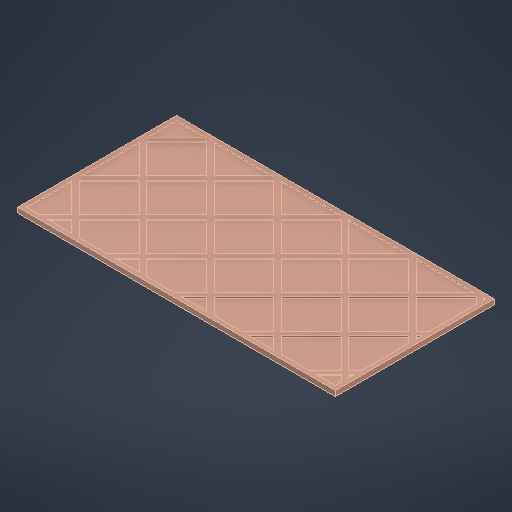
# Autodesk Inventor part: TILE 30X60
Saved by Autodesk Inventor 2025 (Build 290162000, 162)
## iProperties
Created: 2024-05-06
Part Number: TILE 30X60
Material: Generic
Document SubType Name: Modeling
Designer: zulet
Density: 1 g/cm^3
Appearance: Smooth - Dark Brown
Author: zulet
Autodesk Inventor part; units mm, degrees
ref_plane "YZ Plane" through (0, 0, 0) normal (1, 0, 0) x (0, 1, 0)
ref_plane "XZ Plane" through (0, 0, 0) normal (0, 1, 0) x (-1, 0, 0)
ref_plane "XY Plane" through (0, 0, 0) normal (0, 0, 1) x (1, 0, 0)
sketch "Sketch1" plane through (0, 0, 0) normal (0, 1, 0) x (-1, 0, 0)
  line L0 (0, 0) -> (600, 0)
  line L1 (600, 0) -> (600, -300)
  line L2 (600, -300) -> (0, -300)
  line L3 (0, -300) -> (0, 0)
  dimension "d0" = 600
  dimension "d1" = 300
  constraints: 8 end point, 2 parallel, 1 horizontal, 1 perpendicular
  measures "d0" distance of L1.end L2.end
  measures "d1" distance of L0.end L1.end
extrude "Extrusion1" add sketch "Sketch1" along normal blind 8
sketch "Sketch2" plane through (0, 8, 0) normal (0, 1, 0) x (1, 0, 0)
  line L0 (-656.5685, 300) -> (-600, 356.5685)
  line L1 (-600, 356.5685) -> (-656.5685, 413.1371)
  line L2 (-656.5685, 413.1371) -> (-713.1371, 356.5685)
  line L3 (-713.1371, 356.5685) -> (-656.5685, 300)
  line L4 (-656.5685, 300) -> (-656.5685, 413.1371) construction
  line L5 (-600, 356.5685) -> (-713.1371, 356.5685) construction
  line L6 (-656.5685, 300) -> (-576.5685, 300) construction
  line L7 (0, 300) -> (-600, 300) projected
  line L8 (-600, 300) -> (-600, 0) projected
  line L9 (-592.9289, 236.3604) -> (-536.3604, 292.9289)
  line L10 (-536.3604, 292.9289) -> (-592.9289, 349.4975)
  line L11 (-592.9289, 349.4975) -> (-649.4975, 292.9289)
  line L12 (-649.4975, 292.9289) -> (-592.9289, 236.3604)
  line L13 (-592.9289, 236.3604) -> (-592.9289, 349.4975) construction
  line L14 (-536.3604, 292.9289) -> (-649.4975, 292.9289) construction
  line L15 (-529.2893, 172.7208) -> (-472.7208, 229.2893)
  line L16 (-472.7208, 229.2893) -> (-529.2893, 285.8579)
  line L17 (-529.2893, 285.8579) -> (-585.8579, 229.2893)
  line L18 (-585.8579, 229.2893) -> (-529.2893, 172.7208)
  line L19 (-529.2893, 172.7208) -> (-529.2893, 285.8579) construction
  line L20 (-472.7208, 229.2893) -> (-585.8579, 229.2893) construction
  line L21 (-465.6497, 109.0812) -> (-409.0812, 165.6497)
  line L22 (-409.0812, 165.6497) -> (-465.6497, 222.2183)
  line L23 (-465.6497, 222.2183) -> (-522.2183, 165.6497)
  line L24 (-522.2183, 165.6497) -> (-465.6497, 109.0812)
  line L25 (-465.6497, 109.0812) -> (-465.6497, 222.2183) construction
  line L26 (-409.0812, 165.6497) -> (-522.2183, 165.6497) construction
  line L27 (-402.0101, 45.4416) -> (-345.4416, 102.0101)
  line L28 (-345.4416, 102.0101) -> (-402.0101, 158.5786)
  line L29 (-402.0101, 158.5786) -> (-458.5786, 102.0101)
  line L30 (-458.5786, 102.0101) -> (-402.0101, 45.4416)
  line L31 (-402.0101, 45.4416) -> (-402.0101, 158.5786) construction
  line L32 (-345.4416, 102.0101) -> (-458.5786, 102.0101) construction
  line L33 (-338.3705, -18.1981) -> (-281.8019, 38.3705)
  line L34 (-281.8019, 38.3705) -> (-338.3705, 94.939)
  line L35 (-338.3705, 94.939) -> (-394.939, 38.3705)
  line L36 (-394.939, 38.3705) -> (-338.3705, -18.1981)
  line L37 (-338.3705, -18.1981) -> (-338.3705, 94.939) construction
  line L38 (-281.8019, 38.3705) -> (-394.939, 38.3705) construction
  line L39 (-274.7309, -81.8377) -> (-218.1623, -25.2691)
  line L40 (-218.1623, -25.2691) -> (-274.7309, 31.2994)
  line L41 (-274.7309, 31.2994) -> (-331.2994, -25.2691)
  line L42 (-331.2994, -25.2691) -> (-274.7309, -81.8377)
  line L43 (-274.7309, -81.8377) -> (-274.7309, 31.2994) construction
  line L44 (-218.1623, -25.2691) -> (-331.2994, -25.2691) construction
  line L45 (-211.0913, -145.4773) -> (-154.5227, -88.9087)
  line L46 (-154.5227, -88.9087) -> (-211.0913, -32.3402)
  line L47 (-211.0913, -32.3402) -> (-267.6598, -88.9087)
  line L48 (-267.6598, -88.9087) -> (-211.0913, -145.4773)
  line L49 (-211.0913, -145.4773) -> (-211.0913, -32.3402) construction
  line L50 (-154.5227, -88.9087) -> (-267.6598, -88.9087) construction
  line L51 (-147.4517, -209.1169) -> (-90.8831, -152.5483)
  line L52 (-90.8831, -152.5483) -> (-147.4517, -95.9798)
  line L53 (-147.4517, -95.9798) -> (-204.0202, -152.5483)
  line L54 (-204.0202, -152.5483) -> (-147.4517, -209.1169)
  line L55 (-147.4517, -209.1169) -> (-147.4517, -95.9798) construction
  line L56 (-90.8831, -152.5483) -> (-204.0202, -152.5483) construction
  line L57 (-83.812, -272.7565) -> (-27.2435, -216.188)
  line L58 (-27.2435, -216.188) -> (-83.812, -159.6194)
  line L59 (-83.812, -159.6194) -> (-140.3806, -216.188)
  line L60 (-140.3806, -216.188) -> (-83.812, -272.7565)
  line L61 (-83.812, -272.7565) -> (-83.812, -159.6194) construction
  line L62 (-27.2435, -216.188) -> (-140.3806, -216.188) construction
  line L63 (-592.9289, 363.6396) -> (-536.3604, 420.2082)
  line L64 (-536.3604, 420.2082) -> (-592.9289, 476.7767)
  line L65 (-592.9289, 476.7767) -> (-649.4975, 420.2082)
  line L66 (-649.4975, 420.2082) -> (-592.9289, 363.6396)
  line L67 (-592.9289, 363.6396) -> (-592.9289, 476.7767) construction
  line L68 (-536.3604, 420.2082) -> (-649.4975, 420.2082) construction
  line L69 (-529.2893, 300) -> (-472.7208, 356.5685)
  line L70 (-472.7208, 356.5685) -> (-529.2893, 413.1371)
  line L71 (-529.2893, 413.1371) -> (-585.8579, 356.5685)
  line L72 (-585.8579, 356.5685) -> (-529.2893, 300)
  line L73 (-529.2893, 300) -> (-529.2893, 413.1371) construction
  line L74 (-472.7208, 356.5685) -> (-585.8579, 356.5685) construction
  line L75 (-465.6497, 236.3604) -> (-409.0812, 292.9289)
  line L76 (-409.0812, 292.9289) -> (-465.6497, 349.4975)
  line L77 (-465.6497, 349.4975) -> (-522.2183, 292.9289)
  line L78 (-522.2183, 292.9289) -> (-465.6497, 236.3604)
  line L79 (-465.6497, 236.3604) -> (-465.6497, 349.4975) construction
  line L80 (-409.0812, 292.9289) -> (-522.2183, 292.9289) construction
  line L81 (-402.0101, 172.7208) -> (-345.4416, 229.2893)
  line L82 (-345.4416, 229.2893) -> (-402.0101, 285.8579)
  line L83 (-402.0101, 285.8579) -> (-458.5786, 229.2893)
  line L84 (-458.5786, 229.2893) -> (-402.0101, 172.7208)
  line L85 (-402.0101, 172.7208) -> (-402.0101, 285.8579) construction
  line L86 (-345.4416, 229.2893) -> (-458.5786, 229.2893) construction
  line L87 (-338.3705, 109.0812) -> (-281.8019, 165.6497)
  line L88 (-281.8019, 165.6497) -> (-338.3705, 222.2183)
  line L89 (-338.3705, 222.2183) -> (-394.939, 165.6497)
  line L90 (-394.939, 165.6497) -> (-338.3705, 109.0812)
  line L91 (-338.3705, 109.0812) -> (-338.3705, 222.2183) construction
  line L92 (-281.8019, 165.6497) -> (-394.939, 165.6497) construction
  line L93 (-274.7309, 45.4416) -> (-218.1623, 102.0101)
  line L94 (-218.1623, 102.0101) -> (-274.7309, 158.5786)
  line L95 (-274.7309, 158.5786) -> (-331.2994, 102.0101)
  line L96 (-331.2994, 102.0101) -> (-274.7309, 45.4416)
  line L97 (-274.7309, 45.4416) -> (-274.7309, 158.5786) construction
  line L98 (-218.1623, 102.0101) -> (-331.2994, 102.0101) construction
  line L99 (-211.0913, -18.1981) -> (-154.5227, 38.3705)
  line L100 (-154.5227, 38.3705) -> (-211.0913, 94.939)
  line L101 (-211.0913, 94.939) -> (-267.6598, 38.3705)
  line L102 (-267.6598, 38.3705) -> (-211.0913, -18.1981)
  line L103 (-211.0913, -18.1981) -> (-211.0913, 94.939) construction
  line L104 (-154.5227, 38.3705) -> (-267.6598, 38.3705) construction
  line L105 (-147.4517, -81.8377) -> (-90.8831, -25.2691)
  line L106 (-90.8831, -25.2691) -> (-147.4517, 31.2994)
  line L107 (-147.4517, 31.2994) -> (-204.0202, -25.2691)
  line L108 (-204.0202, -25.2691) -> (-147.4517, -81.8377)
  line L109 (-147.4517, -81.8377) -> (-147.4517, 31.2994) construction
  line L110 (-90.8831, -25.2691) -> (-204.0202, -25.2691) construction
  line L111 (-83.812, -145.4773) -> (-27.2435, -88.9087)
  line L112 (-27.2435, -88.9087) -> (-83.812, -32.3402)
  line L113 (-83.812, -32.3402) -> (-140.3806, -88.9087)
  line L114 (-140.3806, -88.9087) -> (-83.812, -145.4773)
  line L115 (-83.812, -145.4773) -> (-83.812, -32.3402) construction
  line L116 (-27.2435, -88.9087) -> (-140.3806, -88.9087) construction
  line L117 (-20.1724, -209.1169) -> (36.3961, -152.5483)
  line L118 (36.3961, -152.5483) -> (-20.1724, -95.9798)
  line L119 (-20.1724, -95.9798) -> (-76.741, -152.5483)
  line L120 (-76.741, -152.5483) -> (-20.1724, -209.1169)
  line L121 (-20.1724, -209.1169) -> (-20.1724, -95.9798) construction
  line L122 (36.3961, -152.5483) -> (-76.741, -152.5483) construction
  line L123 (-720.2082, 236.3604) -> (-663.6396, 292.9289)
  line L124 (-663.6396, 292.9289) -> (-720.2082, 349.4975)
  line L125 (-720.2082, 349.4975) -> (-776.7767, 292.9289)
  line L126 (-776.7767, 292.9289) -> (-720.2082, 236.3604)
  line L127 (-720.2082, 236.3604) -> (-720.2082, 349.4975) construction
  line L128 (-663.6396, 292.9289) -> (-776.7767, 292.9289) construction
  line L129 (-656.5685, 172.7208) -> (-600, 229.2893)
  line L130 (-600, 229.2893) -> (-656.5685, 285.8579)
  line L131 (-656.5685, 285.8579) -> (-713.1371, 229.2893)
  line L132 (-713.1371, 229.2893) -> (-656.5685, 172.7208)
  line L133 (-656.5685, 172.7208) -> (-656.5685, 285.8579) construction
  line L134 (-600, 229.2893) -> (-713.1371, 229.2893) construction
  line L135 (-592.9289, 109.0812) -> (-536.3604, 165.6497)
  line L136 (-536.3604, 165.6497) -> (-592.9289, 222.2183)
  line L137 (-592.9289, 222.2183) -> (-649.4975, 165.6497)
  line L138 (-649.4975, 165.6497) -> (-592.9289, 109.0812)
  line L139 (-592.9289, 109.0812) -> (-592.9289, 222.2183) construction
  line L140 (-536.3604, 165.6497) -> (-649.4975, 165.6497) construction
  line L141 (-529.2893, 45.4416) -> (-472.7208, 102.0101)
  line L142 (-472.7208, 102.0101) -> (-529.2893, 158.5786)
  line L143 (-529.2893, 158.5786) -> (-585.8579, 102.0101)
  line L144 (-585.8579, 102.0101) -> (-529.2893, 45.4416)
  line L145 (-529.2893, 45.4416) -> (-529.2893, 158.5786) construction
  line L146 (-472.7208, 102.0101) -> (-585.8579, 102.0101) construction
  line L147 (-465.6497, -18.1981) -> (-409.0812, 38.3705)
  line L148 (-409.0812, 38.3705) -> (-465.6497, 94.939)
  line L149 (-465.6497, 94.939) -> (-522.2183, 38.3705)
  line L150 (-522.2183, 38.3705) -> (-465.6497, -18.1981)
  line L151 (-465.6497, -18.1981) -> (-465.6497, 94.939) construction
  line L152 (-409.0812, 38.3705) -> (-522.2183, 38.3705) construction
  line L153 (-402.0101, -81.8377) -> (-345.4416, -25.2691)
  line L154 (-345.4416, -25.2691) -> (-402.0101, 31.2994)
  line L155 (-402.0101, 31.2994) -> (-458.5786, -25.2691)
  line L156 (-458.5786, -25.2691) -> (-402.0101, -81.8377)
  line L157 (-402.0101, -81.8377) -> (-402.0101, 31.2994) construction
  line L158 (-345.4416, -25.2691) -> (-458.5786, -25.2691) construction
  line L159 (-338.3705, -145.4773) -> (-281.8019, -88.9087)
  line L160 (-281.8019, -88.9087) -> (-338.3705, -32.3402)
  line L161 (-338.3705, -32.3402) -> (-394.939, -88.9087)
  line L162 (-394.939, -88.9087) -> (-338.3705, -145.4773)
  line L163 (-338.3705, -145.4773) -> (-338.3705, -32.3402) construction
  line L164 (-281.8019, -88.9087) -> (-394.939, -88.9087) construction
  line L165 (-274.7309, -209.1169) -> (-218.1623, -152.5483)
  line L166 (-218.1623, -152.5483) -> (-274.7309, -95.9798)
  line L167 (-274.7309, -95.9798) -> (-331.2994, -152.5483)
  line L168 (-331.2994, -152.5483) -> (-274.7309, -209.1169)
  line L169 (-274.7309, -209.1169) -> (-274.7309, -95.9798) construction
  line L170 (-218.1623, -152.5483) -> (-331.2994, -152.5483) construction
  line L171 (-211.0913, -272.7565) -> (-154.5227, -216.188)
  line L172 (-154.5227, -216.188) -> (-211.0913, -159.6194)
  line L173 (-211.0913, -159.6194) -> (-267.6598, -216.188)
  line L174 (-267.6598, -216.188) -> (-211.0913, -272.7565)
  line L175 (-211.0913, -272.7565) -> (-211.0913, -159.6194) construction
  line L176 (-154.5227, -216.188) -> (-267.6598, -216.188) construction
  line L177 (-147.4517, -336.3961) -> (-90.8831, -279.8276)
  line L178 (-90.8831, -279.8276) -> (-147.4517, -223.259)
  line L179 (-147.4517, -223.259) -> (-204.0202, -279.8276)
  line L180 (-204.0202, -279.8276) -> (-147.4517, -336.3961)
  line L181 (-147.4517, -336.3961) -> (-147.4517, -223.259) construction
  line L182 (-90.8831, -279.8276) -> (-204.0202, -279.8276) construction
  line L183 (-529.2893, 427.2792) -> (-472.7208, 483.8478)
  line L184 (-472.7208, 483.8478) -> (-529.2893, 540.4163)
  line L185 (-529.2893, 540.4163) -> (-585.8579, 483.8478)
  line L186 (-585.8579, 483.8478) -> (-529.2893, 427.2792)
  line L187 (-529.2893, 427.2792) -> (-529.2893, 540.4163) construction
  line L188 (-472.7208, 483.8478) -> (-585.8579, 483.8478) construction
  line L189 (-465.6497, 363.6396) -> (-409.0812, 420.2082)
  line L190 (-409.0812, 420.2082) -> (-465.6497, 476.7767)
  line L191 (-465.6497, 476.7767) -> (-522.2183, 420.2082)
  line L192 (-522.2183, 420.2082) -> (-465.6497, 363.6396)
  line L193 (-465.6497, 363.6396) -> (-465.6497, 476.7767) construction
  line L194 (-409.0812, 420.2082) -> (-522.2183, 420.2082) construction
  line L195 (-402.0101, 300) -> (-345.4416, 356.5685)
  line L196 (-345.4416, 356.5685) -> (-402.0101, 413.1371)
  line L197 (-402.0101, 413.1371) -> (-458.5786, 356.5685)
  line L198 (-458.5786, 356.5685) -> (-402.0101, 300)
  line L199 (-402.0101, 300) -> (-402.0101, 413.1371) construction
  line L200 (-345.4416, 356.5685) -> (-458.5786, 356.5685) construction
  line L201 (-338.3705, 236.3604) -> (-281.8019, 292.9289)
  line L202 (-281.8019, 292.9289) -> (-338.3705, 349.4975)
  line L203 (-338.3705, 349.4975) -> (-394.939, 292.9289)
  line L204 (-394.939, 292.9289) -> (-338.3705, 236.3604)
  line L205 (-338.3705, 236.3604) -> (-338.3705, 349.4975) construction
  line L206 (-281.8019, 292.9289) -> (-394.939, 292.9289) construction
  line L207 (-274.7309, 172.7208) -> (-218.1623, 229.2893)
  line L208 (-218.1623, 229.2893) -> (-274.7309, 285.8579)
  line L209 (-274.7309, 285.8579) -> (-331.2994, 229.2893)
  line L210 (-331.2994, 229.2893) -> (-274.7309, 172.7208)
  line L211 (-274.7309, 172.7208) -> (-274.7309, 285.8579) construction
  line L212 (-218.1623, 229.2893) -> (-331.2994, 229.2893) construction
  line L213 (-211.0913, 109.0812) -> (-154.5227, 165.6497)
  line L214 (-154.5227, 165.6497) -> (-211.0913, 222.2183)
  line L215 (-211.0913, 222.2183) -> (-267.6598, 165.6497)
  line L216 (-267.6598, 165.6497) -> (-211.0913, 109.0812)
  line L217 (-211.0913, 109.0812) -> (-211.0913, 222.2183) construction
  line L218 (-154.5227, 165.6497) -> (-267.6598, 165.6497) construction
  line L219 (-147.4517, 45.4416) -> (-90.8831, 102.0101)
  line L220 (-90.8831, 102.0101) -> (-147.4517, 158.5786)
  line L221 (-147.4517, 158.5786) -> (-204.0202, 102.0101)
  line L222 (-204.0202, 102.0101) -> (-147.4517, 45.4416)
  line L223 (-147.4517, 45.4416) -> (-147.4517, 158.5786) construction
  line L224 (-90.8831, 102.0101) -> (-204.0202, 102.0101) construction
  line L225 (-83.812, -18.1981) -> (-27.2435, 38.3705)
  line L226 (-27.2435, 38.3705) -> (-83.812, 94.939)
  line L227 (-83.812, 94.939) -> (-140.3806, 38.3705)
  line L228 (-140.3806, 38.3705) -> (-83.812, -18.1981)
  line L229 (-83.812, -18.1981) -> (-83.812, 94.939) construction
  line L230 (-27.2435, 38.3705) -> (-140.3806, 38.3705) construction
  line L231 (-20.1724, -81.8377) -> (36.3961, -25.2691)
  line L232 (36.3961, -25.2691) -> (-20.1724, 31.2994)
  line L233 (-20.1724, 31.2994) -> (-76.741, -25.2691)
  line L234 (-76.741, -25.2691) -> (-20.1724, -81.8377)
  line L235 (-20.1724, -81.8377) -> (-20.1724, 31.2994) construction
  line L236 (36.3961, -25.2691) -> (-76.741, -25.2691) construction
  line L237 (43.4672, -145.4773) -> (100.0357, -88.9087)
  line L238 (100.0357, -88.9087) -> (43.4672, -32.3402)
  line L239 (43.4672, -32.3402) -> (-13.1014, -88.9087)
  line L240 (-13.1014, -88.9087) -> (43.4672, -145.4773)
  line L241 (43.4672, -145.4773) -> (43.4672, -32.3402) construction
  line L242 (100.0357, -88.9087) -> (-13.1014, -88.9087) construction
  line L243 (-783.8478, 172.7208) -> (-727.2792, 229.2893)
  line L244 (-727.2792, 229.2893) -> (-783.8478, 285.8579)
  line L245 (-783.8478, 285.8579) -> (-840.4163, 229.2893)
  line L246 (-840.4163, 229.2893) -> (-783.8478, 172.7208)
  line L247 (-783.8478, 172.7208) -> (-783.8478, 285.8579) construction
  line L248 (-727.2792, 229.2893) -> (-840.4163, 229.2893) construction
  line L249 (-720.2082, 109.0812) -> (-663.6396, 165.6497)
  line L250 (-663.6396, 165.6497) -> (-720.2082, 222.2183)
  line L251 (-720.2082, 222.2183) -> (-776.7767, 165.6497)
  line L252 (-776.7767, 165.6497) -> (-720.2082, 109.0812)
  line L253 (-720.2082, 109.0812) -> (-720.2082, 222.2183) construction
  line L254 (-663.6396, 165.6497) -> (-776.7767, 165.6497) construction
  line L255 (-656.5685, 45.4416) -> (-600, 102.0101)
  line L256 (-600, 102.0101) -> (-656.5685, 158.5786)
  line L257 (-656.5685, 158.5786) -> (-713.1371, 102.0101)
  line L258 (-713.1371, 102.0101) -> (-656.5685, 45.4416)
  line L259 (-656.5685, 45.4416) -> (-656.5685, 158.5786) construction
  line L260 (-600, 102.0101) -> (-713.1371, 102.0101) construction
  line L261 (-592.9289, -18.1981) -> (-536.3604, 38.3705)
  line L262 (-536.3604, 38.3705) -> (-592.9289, 94.939)
  line L263 (-592.9289, 94.939) -> (-649.4975, 38.3705)
  line L264 (-649.4975, 38.3705) -> (-592.9289, -18.1981)
  line L265 (-592.9289, -18.1981) -> (-592.9289, 94.939) construction
  line L266 (-536.3604, 38.3705) -> (-649.4975, 38.3705) construction
  line L267 (-529.2893, -81.8377) -> (-472.7208, -25.2691)
  line L268 (-472.7208, -25.2691) -> (-529.2893, 31.2994)
  line L269 (-529.2893, 31.2994) -> (-585.8579, -25.2691)
  line L270 (-585.8579, -25.2691) -> (-529.2893, -81.8377)
  line L271 (-529.2893, -81.8377) -> (-529.2893, 31.2994) construction
  line L272 (-472.7208, -25.2691) -> (-585.8579, -25.2691) construction
  line L273 (-465.6497, -145.4773) -> (-409.0812, -88.9087)
  line L274 (-409.0812, -88.9087) -> (-465.6497, -32.3402)
  line L275 (-465.6497, -32.3402) -> (-522.2183, -88.9087)
  line L276 (-522.2183, -88.9087) -> (-465.6497, -145.4773)
  line L277 (-465.6497, -145.4773) -> (-465.6497, -32.3402) construction
  line L278 (-409.0812, -88.9087) -> (-522.2183, -88.9087) construction
  line L279 (-402.0101, -209.1169) -> (-345.4416, -152.5483)
  line L280 (-345.4416, -152.5483) -> (-402.0101, -95.9798)
  line L281 (-402.0101, -95.9798) -> (-458.5786, -152.5483)
  line L282 (-458.5786, -152.5483) -> (-402.0101, -209.1169)
  line L283 (-402.0101, -209.1169) -> (-402.0101, -95.9798) construction
  line L284 (-345.4416, -152.5483) -> (-458.5786, -152.5483) construction
  line L285 (-338.3705, -272.7565) -> (-281.8019, -216.188)
  line L286 (-281.8019, -216.188) -> (-338.3705, -159.6194)
  line L287 (-338.3705, -159.6194) -> (-394.939, -216.188)
  line L288 (-394.939, -216.188) -> (-338.3705, -272.7565)
  line L289 (-338.3705, -272.7565) -> (-338.3705, -159.6194) construction
  line L290 (-281.8019, -216.188) -> (-394.939, -216.188) construction
  line L291 (-274.7309, -336.3961) -> (-218.1623, -279.8276)
  line L292 (-218.1623, -279.8276) -> (-274.7309, -223.259)
  line L293 (-274.7309, -223.259) -> (-331.2994, -279.8276)
  line L294 (-331.2994, -279.8276) -> (-274.7309, -336.3961)
  line L295 (-274.7309, -336.3961) -> (-274.7309, -223.259) construction
  line L296 (-218.1623, -279.8276) -> (-331.2994, -279.8276) construction
  line L297 (-211.0913, -400.0357) -> (-154.5227, -343.4672)
  line L298 (-154.5227, -343.4672) -> (-211.0913, -286.8986)
  line L299 (-211.0913, -286.8986) -> (-267.6598, -343.4672)
  line L300 (-267.6598, -343.4672) -> (-211.0913, -400.0357)
  line L301 (-211.0913, -400.0357) -> (-211.0913, -286.8986) construction
  line L302 (-154.5227, -343.4672) -> (-267.6598, -343.4672) construction
  line L303 (-465.6497, 490.9188) -> (-409.0812, 547.4874)
  line L304 (-409.0812, 547.4874) -> (-465.6497, 604.0559)
  line L305 (-465.6497, 604.0559) -> (-522.2183, 547.4874)
  line L306 (-522.2183, 547.4874) -> (-465.6497, 490.9188)
  line L307 (-465.6497, 490.9188) -> (-465.6497, 604.0559) construction
  line L308 (-409.0812, 547.4874) -> (-522.2183, 547.4874) construction
  line L309 (-402.0101, 427.2792) -> (-345.4416, 483.8478)
  line L310 (-345.4416, 483.8478) -> (-402.0101, 540.4163)
  line L311 (-402.0101, 540.4163) -> (-458.5786, 483.8478)
  line L312 (-458.5786, 483.8478) -> (-402.0101, 427.2792)
  line L313 (-402.0101, 427.2792) -> (-402.0101, 540.4163) construction
  line L314 (-345.4416, 483.8478) -> (-458.5786, 483.8478) construction
  line L315 (-338.3705, 363.6396) -> (-281.8019, 420.2082)
  line L316 (-281.8019, 420.2082) -> (-338.3705, 476.7767)
  line L317 (-338.3705, 476.7767) -> (-394.939, 420.2082)
  line L318 (-394.939, 420.2082) -> (-338.3705, 363.6396)
  line L319 (-338.3705, 363.6396) -> (-338.3705, 476.7767) construction
  line L320 (-281.8019, 420.2082) -> (-394.939, 420.2082) construction
  line L321 (-274.7309, 300) -> (-218.1623, 356.5685)
  line L322 (-218.1623, 356.5685) -> (-274.7309, 413.1371)
  line L323 (-274.7309, 413.1371) -> (-331.2994, 356.5685)
  line L324 (-331.2994, 356.5685) -> (-274.7309, 300)
  line L325 (-274.7309, 300) -> (-274.7309, 413.1371) construction
  line L326 (-218.1623, 356.5685) -> (-331.2994, 356.5685) construction
  line L327 (-211.0913, 236.3604) -> (-154.5227, 292.9289)
  line L328 (-154.5227, 292.9289) -> (-211.0913, 349.4975)
  line L329 (-211.0913, 349.4975) -> (-267.6598, 292.9289)
  line L330 (-267.6598, 292.9289) -> (-211.0913, 236.3604)
  line L331 (-211.0913, 236.3604) -> (-211.0913, 349.4975) construction
  line L332 (-154.5227, 292.9289) -> (-267.6598, 292.9289) construction
  line L333 (-147.4517, 172.7208) -> (-90.8831, 229.2893)
  line L334 (-90.8831, 229.2893) -> (-147.4517, 285.8579)
  line L335 (-147.4517, 285.8579) -> (-204.0202, 229.2893)
  line L336 (-204.0202, 229.2893) -> (-147.4517, 172.7208)
  line L337 (-147.4517, 172.7208) -> (-147.4517, 285.8579) construction
  line L338 (-90.8831, 229.2893) -> (-204.0202, 229.2893) construction
  line L339 (-83.812, 109.0812) -> (-27.2435, 165.6497)
  line L340 (-27.2435, 165.6497) -> (-83.812, 222.2183)
  line L341 (-83.812, 222.2183) -> (-140.3806, 165.6497)
  line L342 (-140.3806, 165.6497) -> (-83.812, 109.0812)
  line L343 (-83.812, 109.0812) -> (-83.812, 222.2183) construction
  line L344 (-27.2435, 165.6497) -> (-140.3806, 165.6497) construction
  line L345 (-20.1724, 45.4416) -> (36.3961, 102.0101)
  line L346 (36.3961, 102.0101) -> (-20.1724, 158.5786)
  line L347 (-20.1724, 158.5786) -> (-76.741, 102.0101)
  line L348 (-76.741, 102.0101) -> (-20.1724, 45.4416)
  line L349 (-20.1724, 45.4416) -> (-20.1724, 158.5786) construction
  line L350 (36.3961, 102.0101) -> (-76.741, 102.0101) construction
  line L351 (43.4672, -18.1981) -> (100.0357, 38.3705)
  line L352 (100.0357, 38.3705) -> (43.4672, 94.939)
  line L353 (43.4672, 94.939) -> (-13.1014, 38.3705)
  line L354 (-13.1014, 38.3705) -> (43.4672, -18.1981)
  line L355 (43.4672, -18.1981) -> (43.4672, 94.939) construction
  line L356 (100.0357, 38.3705) -> (-13.1014, 38.3705) construction
  line L357 (107.1068, -81.8377) -> (163.6753, -25.2691)
  line L358 (163.6753, -25.2691) -> (107.1068, 31.2994)
  line L359 (107.1068, 31.2994) -> (50.5382, -25.2691)
  line L360 (50.5382, -25.2691) -> (107.1068, -81.8377)
  line L361 (107.1068, -81.8377) -> (107.1068, 31.2994) construction
  line L362 (163.6753, -25.2691) -> (50.5382, -25.2691) construction
  line L363 (-847.4874, 109.0812) -> (-790.9188, 165.6497)
  line L364 (-790.9188, 165.6497) -> (-847.4874, 222.2183)
  line L365 (-847.4874, 222.2183) -> (-904.0559, 165.6497)
  line L366 (-904.0559, 165.6497) -> (-847.4874, 109.0812)
  line L367 (-847.4874, 109.0812) -> (-847.4874, 222.2183) construction
  line L368 (-790.9188, 165.6497) -> (-904.0559, 165.6497) construction
  line L369 (-783.8478, 45.4416) -> (-727.2792, 102.0101)
  line L370 (-727.2792, 102.0101) -> (-783.8478, 158.5786)
  line L371 (-783.8478, 158.5786) -> (-840.4163, 102.0101)
  line L372 (-840.4163, 102.0101) -> (-783.8478, 45.4416)
  line L373 (-783.8478, 45.4416) -> (-783.8478, 158.5786) construction
  line L374 (-727.2792, 102.0101) -> (-840.4163, 102.0101) construction
  line L375 (-720.2082, -18.1981) -> (-663.6396, 38.3705)
  line L376 (-663.6396, 38.3705) -> (-720.2082, 94.939)
  line L377 (-720.2082, 94.939) -> (-776.7767, 38.3705)
  line L378 (-776.7767, 38.3705) -> (-720.2082, -18.1981)
  line L379 (-720.2082, -18.1981) -> (-720.2082, 94.939) construction
  line L380 (-663.6396, 38.3705) -> (-776.7767, 38.3705) construction
  line L381 (-656.5685, -81.8377) -> (-600, -25.2691)
  line L382 (-600, -25.2691) -> (-656.5685, 31.2994)
  line L383 (-656.5685, 31.2994) -> (-713.1371, -25.2691)
  line L384 (-713.1371, -25.2691) -> (-656.5685, -81.8377)
  line L385 (-656.5685, -81.8377) -> (-656.5685, 31.2994) construction
  line L386 (-600, -25.2691) -> (-713.1371, -25.2691) construction
  line L387 (-592.9289, -145.4773) -> (-536.3604, -88.9087)
  line L388 (-536.3604, -88.9087) -> (-592.9289, -32.3402)
  line L389 (-592.9289, -32.3402) -> (-649.4975, -88.9087)
  line L390 (-649.4975, -88.9087) -> (-592.9289, -145.4773)
  line L391 (-592.9289, -145.4773) -> (-592.9289, -32.3402) construction
  line L392 (-536.3604, -88.9087) -> (-649.4975, -88.9087) construction
  line L393 (-529.2893, -209.1169) -> (-472.7208, -152.5483)
  line L394 (-472.7208, -152.5483) -> (-529.2893, -95.9798)
  line L395 (-529.2893, -95.9798) -> (-585.8579, -152.5483)
  line L396 (-585.8579, -152.5483) -> (-529.2893, -209.1169)
  line L397 (-529.2893, -209.1169) -> (-529.2893, -95.9798) construction
  line L398 (-472.7208, -152.5483) -> (-585.8579, -152.5483) construction
  line L399 (-465.6497, -272.7565) -> (-409.0812, -216.188)
  line L400 (-409.0812, -216.188) -> (-465.6497, -159.6194)
  line L401 (-465.6497, -159.6194) -> (-522.2183, -216.188)
  line L402 (-522.2183, -216.188) -> (-465.6497, -272.7565)
  line L403 (-465.6497, -272.7565) -> (-465.6497, -159.6194) construction
  line L404 (-409.0812, -216.188) -> (-522.2183, -216.188) construction
  line L405 (-402.0101, -336.3961) -> (-345.4416, -279.8276)
  line L406 (-345.4416, -279.8276) -> (-402.0101, -223.259)
  line L407 (-402.0101, -223.259) -> (-458.5786, -279.8276)
  line L408 (-458.5786, -279.8276) -> (-402.0101, -336.3961)
  line L409 (-402.0101, -336.3961) -> (-402.0101, -223.259) construction
  line L410 (-345.4416, -279.8276) -> (-458.5786, -279.8276) construction
  line L411 (-338.3705, -400.0357) -> (-281.8019, -343.4672)
  line L412 (-281.8019, -343.4672) -> (-338.3705, -286.8986)
  line L413 (-338.3705, -286.8986) -> (-394.939, -343.4672)
  line L414 (-394.939, -343.4672) -> (-338.3705, -400.0357)
  line L415 (-338.3705, -400.0357) -> (-338.3705, -286.8986) construction
  line L416 (-281.8019, -343.4672) -> (-394.939, -343.4672) construction
  line L417 (-274.7309, -463.6753) -> (-218.1623, -407.1068)
  line L418 (-218.1623, -407.1068) -> (-274.7309, -350.5382)
  line L419 (-274.7309, -350.5382) -> (-331.2994, -407.1068)
  line L420 (-331.2994, -407.1068) -> (-274.7309, -463.6753)
  line L421 (-274.7309, -463.6753) -> (-274.7309, -350.5382) construction
  line L422 (-218.1623, -407.1068) -> (-331.2994, -407.1068) construction
  line L423 (-402.0101, 554.5584) -> (-345.4416, 611.127)
  line L424 (-345.4416, 611.127) -> (-402.0101, 667.6955)
  line L425 (-402.0101, 667.6955) -> (-458.5786, 611.127)
  line L426 (-458.5786, 611.127) -> (-402.0101, 554.5584)
  line L427 (-402.0101, 554.5584) -> (-402.0101, 667.6955) construction
  line L428 (-345.4416, 611.127) -> (-458.5786, 611.127) construction
  line L429 (-338.3705, 490.9188) -> (-281.8019, 547.4874)
  line L430 (-281.8019, 547.4874) -> (-338.3705, 604.0559)
  line L431 (-338.3705, 604.0559) -> (-394.939, 547.4874)
  line L432 (-394.939, 547.4874) -> (-338.3705, 490.9188)
  line L433 (-338.3705, 490.9188) -> (-338.3705, 604.0559) construction
  line L434 (-281.8019, 547.4874) -> (-394.939, 547.4874) construction
  line L435 (-274.7309, 427.2792) -> (-218.1623, 483.8478)
  line L436 (-218.1623, 483.8478) -> (-274.7309, 540.4163)
  line L437 (-274.7309, 540.4163) -> (-331.2994, 483.8478)
  line L438 (-331.2994, 483.8478) -> (-274.7309, 427.2792)
  line L439 (-274.7309, 427.2792) -> (-274.7309, 540.4163) construction
  line L440 (-218.1623, 483.8478) -> (-331.2994, 483.8478) construction
  line L441 (-211.0913, 363.6396) -> (-154.5227, 420.2082)
  line L442 (-154.5227, 420.2082) -> (-211.0913, 476.7767)
  line L443 (-211.0913, 476.7767) -> (-267.6598, 420.2082)
  line L444 (-267.6598, 420.2082) -> (-211.0913, 363.6396)
  line L445 (-211.0913, 363.6396) -> (-211.0913, 476.7767) construction
  line L446 (-154.5227, 420.2082) -> (-267.6598, 420.2082) construction
  line L447 (-147.4517, 300) -> (-90.8831, 356.5685)
  line L448 (-90.8831, 356.5685) -> (-147.4517, 413.1371)
  line L449 (-147.4517, 413.1371) -> (-204.0202, 356.5685)
  line L450 (-204.0202, 356.5685) -> (-147.4517, 300)
  line L451 (-147.4517, 300) -> (-147.4517, 413.1371) construction
  line L452 (-90.8831, 356.5685) -> (-204.0202, 356.5685) construction
  line L453 (-83.812, 236.3604) -> (-27.2435, 292.9289)
  line L454 (-27.2435, 292.9289) -> (-83.812, 349.4975)
  line L455 (-83.812, 349.4975) -> (-140.3806, 292.9289)
  line L456 (-140.3806, 292.9289) -> (-83.812, 236.3604)
  line L457 (-83.812, 236.3604) -> (-83.812, 349.4975) construction
  line L458 (-27.2435, 292.9289) -> (-140.3806, 292.9289) construction
  line L459 (-20.1724, 172.7208) -> (36.3961, 229.2893)
  line L460 (36.3961, 229.2893) -> (-20.1724, 285.8579)
  line L461 (-20.1724, 285.8579) -> (-76.741, 229.2893)
  line L462 (-76.741, 229.2893) -> (-20.1724, 172.7208)
  line L463 (-20.1724, 172.7208) -> (-20.1724, 285.8579) construction
  line L464 (36.3961, 229.2893) -> (-76.741, 229.2893) construction
  line L465 (43.4672, 109.0812) -> (100.0357, 165.6497)
  line L466 (100.0357, 165.6497) -> (43.4672, 222.2183)
  line L467 (43.4672, 222.2183) -> (-13.1014, 165.6497)
  line L468 (-13.1014, 165.6497) -> (43.4672, 109.0812)
  line L469 (43.4672, 109.0812) -> (43.4672, 222.2183) construction
  line L470 (100.0357, 165.6497) -> (-13.1014, 165.6497) construction
  line L471 (107.1068, 45.4416) -> (163.6753, 102.0101)
  line L472 (163.6753, 102.0101) -> (107.1068, 158.5786)
  line L473 (107.1068, 158.5786) -> (50.5382, 102.0101)
  line L474 (50.5382, 102.0101) -> (107.1068, 45.4416)
  line L475 (107.1068, 45.4416) -> (107.1068, 158.5786) construction
  line L476 (163.6753, 102.0101) -> (50.5382, 102.0101) construction
  line L477 (170.7464, -18.1981) -> (227.3149, 38.3705)
  line L478 (227.3149, 38.3705) -> (170.7464, 94.939)
  line L479 (170.7464, 94.939) -> (114.1778, 38.3705)
  line L480 (114.1778, 38.3705) -> (170.7464, -18.1981)
  line L481 (170.7464, -18.1981) -> (170.7464, 94.939) construction
  line L482 (227.3149, 38.3705) -> (114.1778, 38.3705) construction
  line L483 (-911.127, 45.4416) -> (-854.5584, 102.0101)
  line L484 (-854.5584, 102.0101) -> (-911.127, 158.5786)
  line L485 (-911.127, 158.5786) -> (-967.6955, 102.0101)
  line L486 (-967.6955, 102.0101) -> (-911.127, 45.4416)
  line L487 (-911.127, 45.4416) -> (-911.127, 158.5786) construction
  line L488 (-854.5584, 102.0101) -> (-967.6955, 102.0101) construction
  line L489 (-847.4874, -18.1981) -> (-790.9188, 38.3705)
  line L490 (-790.9188, 38.3705) -> (-847.4874, 94.939)
  line L491 (-847.4874, 94.939) -> (-904.0559, 38.3705)
  line L492 (-904.0559, 38.3705) -> (-847.4874, -18.1981)
  line L493 (-847.4874, -18.1981) -> (-847.4874, 94.939) construction
  line L494 (-790.9188, 38.3705) -> (-904.0559, 38.3705) construction
  line L495 (-783.8478, -81.8377) -> (-727.2792, -25.2691)
  line L496 (-727.2792, -25.2691) -> (-783.8478, 31.2994)
  line L497 (-783.8478, 31.2994) -> (-840.4163, -25.2691)
  line L498 (-840.4163, -25.2691) -> (-783.8478, -81.8377)
  line L499 (-783.8478, -81.8377) -> (-783.8478, 31.2994) construction
  line L500 (-727.2792, -25.2691) -> (-840.4163, -25.2691) construction
  line L501 (-720.2082, -145.4773) -> (-663.6396, -88.9087)
  line L502 (-663.6396, -88.9087) -> (-720.2082, -32.3402)
  line L503 (-720.2082, -32.3402) -> (-776.7767, -88.9087)
  line L504 (-776.7767, -88.9087) -> (-720.2082, -145.4773)
  line L505 (-720.2082, -145.4773) -> (-720.2082, -32.3402) construction
  line L506 (-663.6396, -88.9087) -> (-776.7767, -88.9087) construction
  line L507 (-656.5685, -209.1169) -> (-600, -152.5483)
  line L508 (-600, -152.5483) -> (-656.5685, -95.9798)
  line L509 (-656.5685, -95.9798) -> (-713.1371, -152.5483)
  line L510 (-713.1371, -152.5483) -> (-656.5685, -209.1169)
  line L511 (-656.5685, -209.1169) -> (-656.5685, -95.9798) construction
  line L512 (-600, -152.5483) -> (-713.1371, -152.5483) construction
  line L513 (-592.9289, -272.7565) -> (-536.3604, -216.188)
  line L514 (-536.3604, -216.188) -> (-592.9289, -159.6194)
  line L515 (-592.9289, -159.6194) -> (-649.4975, -216.188)
  line L516 (-649.4975, -216.188) -> (-592.9289, -272.7565)
  line L517 (-592.9289, -272.7565) -> (-592.9289, -159.6194) construction
  line L518 (-536.3604, -216.188) -> (-649.4975, -216.188) construction
  line L519 (-529.2893, -336.3961) -> (-472.7208, -279.8276)
  line L520 (-472.7208, -279.8276) -> (-529.2893, -223.259)
  line L521 (-529.2893, -223.259) -> (-585.8579, -279.8276)
  line L522 (-585.8579, -279.8276) -> (-529.2893, -336.3961)
  line L523 (-529.2893, -336.3961) -> (-529.2893, -223.259) construction
  line L524 (-472.7208, -279.8276) -> (-585.8579, -279.8276) construction
  line L525 (-465.6497, -400.0357) -> (-409.0812, -343.4672)
  line L526 (-409.0812, -343.4672) -> (-465.6497, -286.8986)
  line L527 (-465.6497, -286.8986) -> (-522.2183, -343.4672)
  line L528 (-522.2183, -343.4672) -> (-465.6497, -400.0357)
  line L529 (-465.6497, -400.0357) -> (-465.6497, -286.8986) construction
  line L530 (-409.0812, -343.4672) -> (-522.2183, -343.4672) construction
  line L531 (-402.0101, -463.6753) -> (-345.4416, -407.1068)
  line L532 (-345.4416, -407.1068) -> (-402.0101, -350.5382)
  line L533 (-402.0101, -350.5382) -> (-458.5786, -407.1068)
  line L534 (-458.5786, -407.1068) -> (-402.0101, -463.6753)
  line L535 (-402.0101, -463.6753) -> (-402.0101, -350.5382) construction
  line L536 (-345.4416, -407.1068) -> (-458.5786, -407.1068) construction
  line L537 (-338.3705, -527.3149) -> (-281.8019, -470.7464)
  line L538 (-281.8019, -470.7464) -> (-338.3705, -414.1778)
  line L539 (-338.3705, -414.1778) -> (-394.939, -470.7464)
  line L540 (-394.939, -470.7464) -> (-338.3705, -527.3149)
  line L541 (-338.3705, -527.3149) -> (-338.3705, -414.1778) construction
  line L542 (-281.8019, -470.7464) -> (-394.939, -470.7464) construction
  line L543 (-338.3705, 618.1981) -> (-281.8019, 674.7666)
  line L544 (-281.8019, 674.7666) -> (-338.3705, 731.3351)
  line L545 (-338.3705, 731.3351) -> (-394.939, 674.7666)
  line L546 (-394.939, 674.7666) -> (-338.3705, 618.1981)
  line L547 (-338.3705, 618.1981) -> (-338.3705, 731.3351) construction
  line L548 (-281.8019, 674.7666) -> (-394.939, 674.7666) construction
  line L549 (-274.7309, 554.5584) -> (-218.1623, 611.127)
  line L550 (-218.1623, 611.127) -> (-274.7309, 667.6955)
  line L551 (-274.7309, 667.6955) -> (-331.2994, 611.127)
  line L552 (-331.2994, 611.127) -> (-274.7309, 554.5584)
  line L553 (-274.7309, 554.5584) -> (-274.7309, 667.6955) construction
  line L554 (-218.1623, 611.127) -> (-331.2994, 611.127) construction
  line L555 (-211.0913, 490.9188) -> (-154.5227, 547.4874)
  line L556 (-154.5227, 547.4874) -> (-211.0913, 604.0559)
  line L557 (-211.0913, 604.0559) -> (-267.6598, 547.4874)
  line L558 (-267.6598, 547.4874) -> (-211.0913, 490.9188)
  line L559 (-211.0913, 490.9188) -> (-211.0913, 604.0559) construction
  line L560 (-154.5227, 547.4874) -> (-267.6598, 547.4874) construction
  line L561 (-147.4517, 427.2792) -> (-90.8831, 483.8478)
  line L562 (-90.8831, 483.8478) -> (-147.4517, 540.4163)
  line L563 (-147.4517, 540.4163) -> (-204.0202, 483.8478)
  line L564 (-204.0202, 483.8478) -> (-147.4517, 427.2792)
  line L565 (-147.4517, 427.2792) -> (-147.4517, 540.4163) construction
  line L566 (-90.8831, 483.8478) -> (-204.0202, 483.8478) construction
  line L567 (-83.812, 363.6396) -> (-27.2435, 420.2082)
  line L568 (-27.2435, 420.2082) -> (-83.812, 476.7767)
  line L569 (-83.812, 476.7767) -> (-140.3806, 420.2082)
  line L570 (-140.3806, 420.2082) -> (-83.812, 363.6396)
  line L571 (-83.812, 363.6396) -> (-83.812, 476.7767) construction
  line L572 (-27.2435, 420.2082) -> (-140.3806, 420.2082) construction
  line L573 (-20.1724, 300) -> (36.3961, 356.5685)
  line L574 (36.3961, 356.5685) -> (-20.1724, 413.1371)
  line L575 (-20.1724, 413.1371) -> (-76.741, 356.5685)
  line L576 (-76.741, 356.5685) -> (-20.1724, 300)
  line L577 (-20.1724, 300) -> (-20.1724, 413.1371) construction
  line L578 (36.3961, 356.5685) -> (-76.741, 356.5685) construction
  line L579 (43.4672, 236.3604) -> (100.0357, 292.9289)
  line L580 (100.0357, 292.9289) -> (43.4672, 349.4975)
  line L581 (43.4672, 349.4975) -> (-13.1014, 292.9289)
  line L582 (-13.1014, 292.9289) -> (43.4672, 236.3604)
  line L583 (43.4672, 236.3604) -> (43.4672, 349.4975) construction
  line L584 (100.0357, 292.9289) -> (-13.1014, 292.9289) construction
  line L585 (107.1068, 172.7208) -> (163.6753, 229.2893)
  line L586 (163.6753, 229.2893) -> (107.1068, 285.8579)
  line L587 (107.1068, 285.8579) -> (50.5382, 229.2893)
  line L588 (50.5382, 229.2893) -> (107.1068, 172.7208)
  line L589 (107.1068, 172.7208) -> (107.1068, 285.8579) construction
  line L590 (163.6753, 229.2893) -> (50.5382, 229.2893) construction
  line L591 (170.7464, 109.0812) -> (227.3149, 165.6497)
  line L592 (227.3149, 165.6497) -> (170.7464, 222.2183)
  line L593 (170.7464, 222.2183) -> (114.1778, 165.6497)
  line L594 (114.1778, 165.6497) -> (170.7464, 109.0812)
  line L595 (170.7464, 109.0812) -> (170.7464, 222.2183) construction
  line L596 (227.3149, 165.6497) -> (114.1778, 165.6497) construction
  line L597 (234.386, 45.4416) -> (290.9545, 102.0101)
  line L598 (290.9545, 102.0101) -> (234.386, 158.5786)
  line L599 (234.386, 158.5786) -> (177.8175, 102.0101)
  line L600 (177.8175, 102.0101) -> (234.386, 45.4416)
  line L601 (234.386, 45.4416) -> (234.386, 158.5786) construction
  line L602 (290.9545, 102.0101) -> (177.8175, 102.0101) construction
  line L603 (0, 300) -> (-600, 300) projected
  line L604 (-600, 300) -> (-600, 0) projected
  line L605 (-600, 0) -> (0, 0) projected
  line L606 (0, 0) -> (0, 300) projected
  line L607 (-8, 8) -> (-592, 8)
  line L608 (-592, 8) -> (-592, 292)
  line L609 (-592, 292) -> (-8, 292)
  line L610 (-8, 292) -> (-8, 8)
  line L611 (-592, 237.2893) -> (-592.9289, 236.3604)
  line L612 (-592.9289, 236.3604) -> (-600, 243.4315)
  line L613 (-600, 243.4315) -> (-600, 300)
  line L614 (-600, 300) -> (-543.4315, 300)
  line L615 (-543.4315, 300) -> (-536.3604, 292.9289)
  line L616 (-536.3604, 292.9289) -> (-537.2893, 292)
  line L617 (-537.2893, 292) -> (-592, 292)
  line L618 (-592, 292) -> (-592, 237.2893)
  point P0 (-656.5685, 356.5685)
  point P1 (-592.9289, 292.9289)
  point P2 (-512.9289, 236.3604)
  point P3 (-529.2893, 229.2893)
  point P4 (-449.2893, 172.7208)
  point P5 (-465.6497, 165.6497)
  point P6 (-385.6497, 109.0812)
  point P7 (-402.0101, 102.0101)
  point P8 (-322.0101, 45.4416)
  point P9 (-338.3705, 38.3705)
  point P10 (-258.3705, -18.1981)
  point P11 (-274.7309, -25.2691)
  point P12 (-194.7309, -81.8377)
  point P13 (-211.0913, -88.9087)
  point P14 (-131.0913, -145.4773)
  point P15 (-147.4517, -152.5483)
  point P16 (-67.4517, -209.1169)
  point P17 (-83.812, -216.188)
  point P18 (-3.812, -272.7565)
  point P19 (-592.9289, 420.2082)
  point P20 (-512.9289, 363.6396)
  point P21 (-529.2893, 356.5685)
  point P22 (-449.2893, 300)
  point P23 (-465.6497, 292.9289)
  point P24 (-385.6497, 236.3604)
  point P25 (-402.0101, 229.2893)
  point P26 (-322.0101, 172.7208)
  point P27 (-338.3705, 165.6497)
  point P28 (-258.3705, 109.0812)
  point P29 (-274.7309, 102.0101)
  point P30 (-194.7309, 45.4416)
  point P31 (-211.0913, 38.3705)
  point P32 (-131.0913, -18.1981)
  point P33 (-147.4517, -25.2691)
  point P34 (-67.4517, -81.8377)
  point P35 (-83.812, -88.9087)
  point P36 (-3.812, -145.4773)
  point P37 (-20.1724, -152.5483)
  point P38 (59.8276, -209.1169)
  point P39 (-720.2082, 292.9289)
  point P40 (-640.2082, 236.3604)
  point P41 (-656.5685, 229.2893)
  point P42 (-576.5685, 172.7208)
  point P43 (-592.9289, 165.6497)
  point P44 (-512.9289, 109.0812)
  point P45 (-529.2893, 102.0101)
  point P46 (-449.2893, 45.4416)
  point P47 (-465.6497, 38.3705)
  point P48 (-385.6497, -18.1981)
  point P49 (-402.0101, -25.2691)
  point P50 (-322.0101, -81.8377)
  point P51 (-338.3705, -88.9087)
  point P52 (-258.3705, -145.4773)
  point P53 (-274.7309, -152.5483)
  point P54 (-194.7309, -209.1169)
  point P55 (-211.0913, -216.188)
  point P56 (-131.0913, -272.7565)
  point P57 (-147.4517, -279.8276)
  point P58 (-67.4517, -336.3961)
  point P59 (-529.2893, 483.8478)
  point P60 (-449.2893, 427.2792)
  point P61 (-465.6497, 420.2082)
  point P62 (-385.6497, 363.6396)
  point P63 (-402.0101, 356.5685)
  point P64 (-322.0101, 300)
  point P65 (-338.3705, 292.9289)
  point P66 (-258.3705, 236.3604)
  point P67 (-274.7309, 229.2893)
  point P68 (-194.7309, 172.7208)
  point P69 (-211.0913, 165.6497)
  point P70 (-131.0913, 109.0812)
  point P71 (-147.4517, 102.0101)
  point P72 (-67.4517, 45.4416)
  point P73 (-83.812, 38.3705)
  point P74 (-3.812, -18.1981)
  point P75 (-20.1724, -25.2691)
  point P76 (59.8276, -81.8377)
  point P77 (43.4672, -88.9087)
  point P78 (123.4672, -145.4773)
  point P79 (-783.8478, 229.2893)
  point P80 (-703.8478, 172.7208)
  point P81 (-720.2082, 165.6497)
  point P82 (-640.2082, 109.0812)
  point P83 (-656.5685, 102.0101)
  point P84 (-576.5685, 45.4416)
  point P85 (-592.9289, 38.3705)
  point P86 (-512.9289, -18.1981)
  point P87 (-529.2893, -25.2691)
  point P88 (-449.2893, -81.8377)
  point P89 (-465.6497, -88.9087)
  point P90 (-385.6497, -145.4773)
  point P91 (-402.0101, -152.5483)
  point P92 (-322.0101, -209.1169)
  point P93 (-338.3705, -216.188)
  point P94 (-258.3705, -272.7565)
  point P95 (-274.7309, -279.8276)
  point P96 (-194.7309, -336.3961)
  point P97 (-211.0913, -343.4672)
  point P98 (-131.0913, -400.0357)
  point P99 (-465.6497, 547.4874)
  point P100 (-385.6497, 490.9188)
  point P101 (-402.0101, 483.8478)
  point P102 (-322.0101, 427.2792)
  point P103 (-338.3705, 420.2082)
  point P104 (-258.3705, 363.6396)
  point P105 (-274.7309, 356.5685)
  point P106 (-194.7309, 300)
  point P107 (-211.0913, 292.9289)
  point P108 (-131.0913, 236.3604)
  point P109 (-147.4517, 229.2893)
  point P110 (-67.4517, 172.7208)
  point P111 (-83.812, 165.6497)
  point P112 (-3.812, 109.0812)
  point P113 (-20.1724, 102.0101)
  point P114 (59.8276, 45.4416)
  point P115 (43.4672, 38.3705)
  point P116 (123.4672, -18.1981)
  point P117 (107.1068, -25.2691)
  point P118 (187.1068, -81.8377)
  point P119 (-847.4874, 165.6497)
  point P120 (-767.4874, 109.0812)
  point P121 (-783.8478, 102.0101)
  point P122 (-703.8478, 45.4416)
  point P123 (-720.2082, 38.3705)
  point P124 (-640.2082, -18.1981)
  point P125 (-656.5685, -25.2691)
  point P126 (-576.5685, -81.8377)
  point P127 (-592.9289, -88.9087)
  point P128 (-512.9289, -145.4773)
  point P129 (-529.2893, -152.5483)
  point P130 (-449.2893, -209.1169)
  point P131 (-465.6497, -216.188)
  point P132 (-385.6497, -272.7565)
  point P133 (-402.0101, -279.8276)
  point P134 (-322.0101, -336.3961)
  point P135 (-338.3705, -343.4672)
  point P136 (-258.3705, -400.0357)
  point P137 (-274.7309, -407.1068)
  point P138 (-194.7309, -463.6753)
  point P139 (-402.0101, 611.127)
  point P140 (-322.0101, 554.5584)
  point P141 (-338.3705, 547.4874)
  point P142 (-258.3705, 490.9188)
  point P143 (-274.7309, 483.8478)
  point P144 (-194.7309, 427.2792)
  point P145 (-211.0913, 420.2082)
  point P146 (-131.0913, 363.6396)
  point P147 (-147.4517, 356.5685)
  point P148 (-67.4517, 300)
  point P149 (-83.812, 292.9289)
  point P150 (-3.812, 236.3604)
  point P151 (-20.1724, 229.2893)
  point P152 (59.8276, 172.7208)
  point P153 (43.4672, 165.6497)
  point P154 (123.4672, 109.0812)
  point P155 (107.1068, 102.0101)
  point P156 (187.1068, 45.4416)
  point P157 (170.7464, 38.3705)
  point P158 (250.7464, -18.1981)
  point P159 (-911.127, 102.0101)
  point P160 (-831.127, 45.4416)
  point P161 (-847.4874, 38.3705)
  point P162 (-767.4874, -18.1981)
  point P163 (-783.8478, -25.2691)
  point P164 (-703.8478, -81.8377)
  point P165 (-720.2082, -88.9087)
  point P166 (-640.2082, -145.4773)
  point P167 (-656.5685, -152.5483)
  point P168 (-576.5685, -209.1169)
  point P169 (-592.9289, -216.188)
  point P170 (-512.9289, -272.7565)
  point P171 (-529.2893, -279.8276)
  point P172 (-449.2893, -336.3961)
  point P173 (-465.6497, -343.4672)
  point P174 (-385.6497, -400.0357)
  point P175 (-402.0101, -407.1068)
  point P176 (-322.0101, -463.6753)
  point P177 (-338.3705, -470.7464)
  point P178 (-258.3705, -527.3149)
  point P179 (-338.3705, 674.7666)
  point P180 (-258.3705, 618.1981)
  point P181 (-274.7309, 611.127)
  point P182 (-194.7309, 554.5584)
  point P183 (-211.0913, 547.4874)
  point P184 (-131.0913, 490.9188)
  point P185 (-147.4517, 483.8478)
  point P186 (-67.4517, 427.2792)
  point P187 (-83.812, 420.2082)
  point P188 (-3.812, 363.6396)
  point P189 (-20.1724, 356.5685)
  point P190 (59.8276, 300)
  point P191 (43.4672, 292.9289)
  point P192 (123.4672, 236.3604)
  point P193 (107.1068, 229.2893)
  point P194 (187.1068, 172.7208)
  point P195 (170.7464, 165.6497)
  point P196 (250.7464, 109.0812)
  point P197 (234.386, 102.0101)
  point P198 (314.386, 45.4416)
  point P199 (-600, 215.1472)
  dimension "d4" = 80
  dimension "d5" = 45
  dimension "d6" = 80
  dimension "d9" = 90
  dimension "d12" = 90
  constraints: 1224 end point, 200 midpoint, 10 point on line, 3 collinear, 3 parallel, 3 perpendicular, 1 equal length, 1 horizontal, 1194 other
  measures "d4" distance of L0.start L0.end
  measures "d5" angle of L6 L0
  measures "d6" distance of L1.end L0.end
  measures "d9" distance of L0.start L9.start
  measures "d12" distance of L0.start L63.start
extrude "Extrusion2" add sketch "Sketch2" along normal blind 2 contours L7 L77 L78 L609 L9 L10 | L10 L9 L609 L608 L12 L8 L7 | L7 L76 L75 L609 L78 L77 | L7 L203 L204 L609 L75 L76 | L12 L9 L608 L136 L137 L8 | L609 L78 L75 L204 L201 L330 L327 L456 L453 L582 L610 L460 L461 L462 L459 L467 L468 L346 L347 L348 L345 L353 L354 L232 L233 L607 L225 L226 L227 L228 L106 L107 L99 L100 L101 L102 L40 L41 L33 L34 L35 L36 L154 L155 L147 L148 L149 L150 L268 L269 L261 L262 L608 L135 L136 L9 | L7 L202 L201 L609 L204 L203 | L137 L136 L608 L135 L138 L8 | L7 L329 L330 L609 L201 L202 | L138 L135 L608 L262 L263 L8 | L608 L607 L261 L605 L8 L263 L262 | L7 L328 L327 L609 L330 L329 | L7 L455 L456 L609 L327 L328 | L607 L269 L605 L261 | L456 L455 L7 L454 L453 L609 | L607 L268 L605 L269 | L453 L454 L7 L581 L582 L609 | L607 L150 L605 L268 | L582 L581 L7 L606 L610 L609 | L607 L147 L605 L150 | L582 L606 L460 L610 | L607 L155 L605 L147 | L460 L606 L459 L610 | L607 L154 L605 L155 | L459 L606 L467 L610 | L607 L36 L605 L154 | L467 L606 L468 L610 | L607 L33 L605 L36 | L468 L606 L346 L610 | L607 L41 L605 L33 | L346 L606 L345 L610 | L607 L40 L605 L41 | L345 L606 L353 L610 | L607 L102 L605 L40 | L353 L606 L354 L610 | L607 L99 L605 L102 | L354 L606 L232 L610 | L607 L107 L605 L99 | L232 L606 L605 L233 L607 L610 | L607 L106 L605 L107 | L607 L228 L605 L106 | L233 L605 L225 L607 | L607 L225 L605 L228
body "Solid1"
